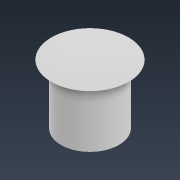
# Autodesk Inventor part: Part3pasador
Saved by Autodesk Inventor 2021.2 (Build 252289000, 289)
## iProperties
Created: 2026-09-01
Part Number: Part3pasador
Material: Generic
Document SubType Name: Modeling
Designer: Tecnica
Density: 1 g/cm^3
Appearance: Default
Author: Tecnica
Autodesk Inventor part; units mm, degrees
ref_plane "YZ Plane" through (0, 0, 0) normal (1, 0, 0) x (0, 1, 0)
ref_plane "XZ Plane" through (0, 0, 0) normal (0, 1, 0) x (-1, 0, 0)
ref_plane "XY Plane" through (0, 0, 0) normal (0, 0, 1) x (1, 0, 0)
sketch "Sketch1" plane through (0, 0, 0) normal (0, 1, 0) x (-1, 0, 0)
  circle A0 centre (0, 0) radius 4.875
  dimension "d0" = 9.75
  constraints: 1 centre point, 1 coincident
  measures "d0" diameter of A0
extrude "Extrusion1" add sketch "Sketch1" along normal blind 10
sketch "Sketch2" plane through (0, 0, 0) normal (1, 0, 0) x (0, 1, 0)
  line L0 (0, 0) -> (10, 0)
  line L1 (10, -4.875) -> (10, 4.875) projected
  line L2 (10, 0) -> (10, -6.5)
  arc A0 (10, -6.5) -> (11.1461, 0) centre (-6.6723, -0.2092) ccw
  line L3 (10, -6.5) -> (11.1461, 0) construction
  line L4 (10, -6.5) -> (16.6003, -6.5) construction
  line L5 (0, -4.875) -> (10, -4.875) projected
  arc A1 (9.4085, -4.875) -> (10, -6.5) centre (13.9141, -4.1553) ccw
  line L6 (10, -6.5) -> (9.4085, -4.875) construction
  line L7 (10, -6.5) -> (11.7293, -6.5) construction
  line L8 (9.4085, -4.875) -> (9.4085, 0)
  line L9 (11.1461, 0) -> (9.4085, 0)
  line L10 (11.1461, 0) -> (0, 0)
  line L11 (0, -4.875) -> (0, 4.875) projected
  dimension "d8" = 6.5
  dimension "d9" = 80
  dimension "d10" = 110
  constraints: 18 end point, 4 point on circle, 3 point on line, 2 centre point, 2 equal length, 2 horizontal, 2 perpendicular, 1 collinear, 1 midpoint
  measures "d8" distance of L0.end L2.end
  measures "d9" angle of L4 L3
  measures "d10" angle of L7 L6
revolve "Revolution1" add sketch "Sketch2" angle 360 about axis through (0, 0, 0) along (0, 1, 0) contours L9 A0 L2 L1 | L5 L2 A1
sketch "Sketch4" plane through (0, 0, 0) normal (0, -1, 0) x (1, 0, 0)
  circle A0 centre (0, 0) radius 1
  dimension "d11" = 2
  constraints: 1 centre point, 1 coincident
  measures "d11" diameter of A0
extrude "Extrusion2" cut sketch "Sketch4" against normal blind 4.5
body "Solid1"
